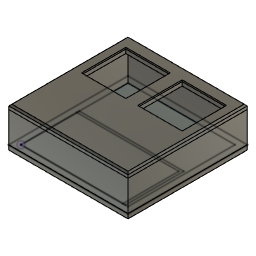
Keypad_Nogap_V2.5L (Autodesk Fusion 360 design; units mm, degrees)
Autodesk Fusion 360 part; units mm, degrees
sketch "Sketch1" plane through (0, 0, 0) normal (0, 0, 1) x (1, 0, 0) in component "case"
  line L0 (0, 0) -> (33.33, 0)
  line L1 (33.33, 0) -> (33.33, 18.3)
  line L2 (33.33, 18.3) -> (0, 18.3)
  line L3 (0, 18.3) -> (0, 0)
  line L4 (34.13, 0) -> (34.13, 19.1)
  line L5 (34.13, 19.1) -> (0, 19.1)
  line L6 (34.13, 0) -> (33.33, 0)
  line L7 (0, 19.1) -> (0, 18.3)
  line L8 (0, 0) -> (35, 0)
  line L9 (35, 0) -> (35, 35)
  line L10 (35, 35) -> (0, 35)
  line L11 (0, 35) -> (0, 0)
  line L12 (-2, 37) -> (-2, -2)
  line L13 (-2, -2) -> (37, -2)
  line L14 (37, -2) -> (37, 37)
  line L15 (37, 37) -> (-2, 37)
  dimension "d1" = 33.33
  dimension "d2" = 18.3
  dimension "d3" = 0.8
  dimension "d4" = 35
  dimension "d5" = 35
  dimension "d6" = 2
  constraint horizontal L0
  constraint vertical L1
  constraint horizontal L2
  constraint vertical L3
  constraint coincident L0.start L3.end
  constraint perpendicular L1 L6
  constraint perpendicular L2 L7
  constraint horizontal L8
  constraint vertical L9
  constraint horizontal L10
  constraint vertical L11
  measures "d1" distance of L0.start L0.end
  measures "d2" distance of L0.start L2.end
  measures "d4" distance of L0.start L8.end
  measures "d5" distance of L0.start L10.end
extrude "Extrude1" add sketch "Sketch1" against normal blind 2 contours L0 L1 L2 L3 L8 L11 | L1 L2 L4 L5 L6 L7 L8 L11 | L4 L5 L8 L9 L10 L11 | L12 L13 L14 L15 makes body 1 in component "case"
extrude "Extrude2" add sketch "Sketch1" along normal blind 1.7 contours L1 L2 L4 L5 L6 L7 L8 L11 bodies 1 in component "case"
ref_plane "WorkPlane1" through (17.5, 17.5, 1.7) normal (0, 0, 1) x (1, 0, 0) in component "case"
extrude "Extrude3" add sketch "Sketch1" along normal blind 10 bodies 1 in component "case"
chamfer "Chamfer1" distance 0.5 angle 45 2 edges at (17.065, 19.1, 0) (34.13, 9.55, 0) on bodies 1 in component "case"
sketch "Sketch2" plane through (17.5, 17.5, 1.7) normal (0, 0, 1) x (1, 0, 0) in component "case"
  line L0 (-17.5, -17.5) -> (15.83, -17.5)
  line L1 (15.83, -17.5) -> (15.83, 0.8)
  line L2 (15.83, 0.8) -> (-17.5, 0.8)
  line L3 (-17.5, 0.8) -> (-17.5, -17.5)
  line L4 (-17.5, -17.5) -> (-17.5, -12.25) construction
  line L5 (-17.5, -12.25) -> (-20, -12.25)
  line L6 (-20, -12.25) -> (-20, -4.75)
  line L7 (-20, -4.75) -> (-17.5, -4.75)
  line L8 (-17.5, -4.75) -> (-17.5, -12.25)
  dimension "d15" = 5.25
  dimension "d16" = 2.5
  dimension "d17" = 7.5
  constraint coincident L0.start L3.end
  constraint perpendicular L0 L4
  constraint horizontal L5
  constraint vertical L6
  constraint horizontal L7
  constraint vertical L8
  measures "d15" distance of L0.start L4.end
  measures "d16" distance of L4.end L5.end
  measures "d17" distance of L4.end L7.end
extrude "Extrude4" cut sketch "Sketch2" along normal blind 2.6 and the other way blind 0.1 contours L3 L5 L6 L7 L8 bodies 1 in component "case"
chamfer "Chamfer2" distance 1 angle 45 2 edges at (-1, 12.75, 1.6) (-1, 5.25, 1.6) on bodies 1 in component "case"
sketch "Sketch3" plane through (-2, 0, 0) normal (-1, 0, 0) x (0, -1, 0) in component "case"
  line L0 (-6.25, 1.6) -> (-11.75, 1.6)
  line L1 (-11.75, 1.6) -> (-12.75, 2.6)
  line L2 (-12.75, 2.6) -> (-12.75, 4.3)
  line L3 (-12.75, 4.3) -> (-5.25, 4.3)
  line L4 (-5.25, 4.3) -> (-5.25, 2.6)
  line L5 (-5.25, 2.6) -> (-6.25, 1.6)
  line L6 (-37, 10) -> (-37, -2)
  line L7 (-37, -2) -> (2, -2)
  line L8 (2, -2) -> (2, 10)
  line L9 (2, 10) -> (-37, 10)
  line L10 (-4.25, 2.1858) -> (-5.8358, 0.6)
  line L11 (-5.8358, 0.6) -> (-12.1642, 0.6)
  line L12 (-12.1642, 0.6) -> (-13.75, 2.1858)
  line L13 (-13.75, 2.1858) -> (-13.75, 5.3)
  line L14 (-13.75, 5.3) -> (-4.25, 5.3)
  line L15 (-4.25, 5.3) -> (-4.25, 2.1858)
  dimension "d23" = -1
  measures "d23" distance of L5
extrude "Extrude5" cut sketch "Sketch3" against normal blind 0.5 contours L10 L11 L12 L13 L14 L15 bodies 1 in component "case"
fillet "Fillet1" radius 0.5 12 edges at (-1.5, 12.9571, 1.3929) (-2, 12.9571, 1.3929) (-2, 13.75, 3.7429) (-1.5, 13.75, 3.7429) (-1.5, 9, 0.6) (-2, 9, 0.6) (-1.5, 9, 5.3) (-2, 9, 5.3) (-1.5, 4.25, 3.7429) (-2, 4.25, 3.7429) (-1.5, 5.0429, 1.3929) (-2, 5.0429, 1.3929) on bodies 1 in component "case"
sketch "Sketch4" plane through (0, 0, 10) normal (0, 0, 1) x (-1, 0, 0) in component "case"
  line L0 (0, 0) -> (0, -35)
  line L1 (0, -35) -> (-35, -35)
  line L2 (-35, -35) -> (-35, 0)
  line L3 (-35, 0) -> (0, 0)
  line L4 (-37, -37) -> (2, -37)
  line L5 (2, -37) -> (2, 2)
  line L6 (2, 2) -> (-37, 2)
  line L7 (-37, 2) -> (-37, -37)
  line L8 (0.8, 0.8) -> (0.8, -35.8)
  line L9 (0.8, -35.8) -> (-35.8, -35.8)
  line L10 (-35.8, -35.8) -> (-35.8, 0.8)
  line L11 (-35.8, 0.8) -> (0.8, 0.8)
  dimension "d28" = -0.8
extrude "Extrude6" cut sketch "Sketch4" against normal blind 1 contours L8 L9 L10 L11 bodies 1 in component "case"
sketch "Sketch1 (2)" plane through (0, 0, 10) normal (0, 0, 1) x (-1, 0, 0) in component "lid"
  line L0 (0.8, -35.8) -> (-35.8, -35.8)
  line L1 (-35.8, -35.8) -> (-35.8, 0.8)
  line L2 (-35.8, 0.8) -> (0.8, 0.8)
  line L3 (0.8, 0.8) -> (0.8, -35.8)
  line L4 (-37, -37) -> (2, -37)
  line L5 (2, -37) -> (2, 2)
  line L6 (2, 2) -> (-37, 2)
  line L7 (-37, 2) -> (-37, -37)
  line L8 (-35, -35) -> (-35, 0)
  line L9 (-35, 0) -> (0, 0)
  line L10 (0, 0) -> (0, -35)
  line L11 (0, -35) -> (-35, -35)
  line L12 (-35.8, 0.8) -> (-35.8, -35.8)
  line L13 (-35.8, -35.8) -> (0.8, -35.8)
  line L14 (0.8, -35.8) -> (0.8, 0.8)
  line L15 (0.8, 0.8) -> (-35.8, 0.8)
  line L16 (0.7, 0.7) -> (0.7, -35.7)
  line L17 (0.7, -35.7) -> (-35.7, -35.7)
  line L18 (-35.7, -35.7) -> (-35.7, 0.7)
  line L19 (-35.7, 0.7) -> (0.7, 0.7)
  dimension "d31" = 0.1
extrude "Extrude1'" add sketch "Sketch1 (2)" against normal blind 0.9 separate body contours L16 L17 L18 L19 makes body 2 in component "lid"
sketch "Sketch2 (2)" plane through (0, 0, 10) normal (0, 0, 1) x (-1, 0, 0) in component "lid"
  line L0 (0.8, -35.8) -> (-35.8, -35.8)
  line L1 (-35.8, -35.8) -> (-35.8, 0.8)
  line L2 (-35.8, 0.8) -> (0.8, 0.8)
  line L3 (0.8, 0.8) -> (0.8, -35.8)
  line L4 (-37, -37) -> (2, -37)
  line L5 (2, -37) -> (2, 2)
  line L6 (2, 2) -> (-37, 2)
  line L7 (-37, 2) -> (-37, -37)
  line L8 (-37, -37) -> (2, -37)
  line L9 (2, -37) -> (2, 2)
  line L10 (2, 2) -> (-37, 2)
  line L11 (-37, 2) -> (-37, -37)
  constraint horizontal L8
  constraint vertical L9
  constraint horizontal L10
  constraint vertical L11
  constraint coincident L5.end L6.start
  constraint coincident L4.start L7.end
extrude "Extrude2'" add sketch "Sketch2 (2)" along normal blind 1.5 contours L0 L1 L2 L3 | L4 L5 L6 L7 L8 L9 L10 L11 bodies 2 in component "lid"
sketch "Sketch3 (2)" plane through (0, 0, 11.5) normal (0, 0, 1) x (-1, 0, 0) in component "lid"
  line L0 (-37, 2) -> (-37, -37)
  line L1 (-37, -37) -> (2, -37)
  line L2 (2, -37) -> (2, 2)
  line L3 (2, 2) -> (-37, 2)
  line L4 (-1.2835, -33) -> (-15.2835, -33)
  line L5 (-15.2835, -33) -> (-15.2835, -19)
  line L6 (-15.2835, -19) -> (-1.2835, -19)
  line L7 (-1.2835, -19) -> (-1.2835, -33)
  line L8 (-15.2835, -19) -> (-19.7168, -19) construction
  line L9 (-19.7168, -19) -> (-33.7168, -19)
  line L10 (-33.7168, -19) -> (-33.7168, -33)
  line L11 (-33.7168, -33) -> (-19.7168, -33)
  line L12 (-19.7168, -33) -> (-19.7168, -19)
  line L13 (-35, -35) -> (-35, 0)
  line L14 (-35, 0) -> (0, 0)
  line L15 (0, 0) -> (0, -35)
  line L16 (0, -35) -> (-35, -35)
  line L17 (-35.8, 0.8) -> (-35.8, -35.8)
  line L18 (-35.8, -35.8) -> (0.8, -35.8)
  line L19 (0.8, -35.8) -> (0.8, 0.8)
  line L20 (0.8, 0.8) -> (-35.8, 0.8)
  line L21 (0.8, -35.8) -> (-35.8, -35.8)
  line L22 (-35.8, -35.8) -> (-35.8, 0.8)
  line L23 (-35.8, 0.8) -> (0.8, 0.8)
  line L24 (0.8, 0.8) -> (0.8, -35.8)
  line L25 (-37, -37) -> (2, -37)
  line L26 (2, -37) -> (2, 2)
  line L27 (2, 2) -> (-37, 2)
  line L28 (-37, 2) -> (-37, -37)
  line L29 (0.8, -26.6121) -> (-1.2835, -26.6121) construction
  line L30 (-6.7358, -33) -> (-6.7358, -35) construction
  dimension "d36" = 14
  dimension "d37" = 14
  dimension "d38" = 4.4333
  dimension "d39" = 14
  dimension "d40" = 14
  dimension "d45" = 2.0835
  constraint horizontal L4
  constraint vertical L5
  constraint horizontal L6
  constraint vertical L7
  constraint perpendicular L5 L8
  constraint horizontal L9
  constraint vertical L10
  constraint horizontal L11
  constraint vertical L12
  constraint coincident L24 L29.start
  constraint coincident L7 L29.end
  constraint perpendicular L7 L29
  constraint coincident L4 L30.start
  constraint coincident L16 L30.end
  constraint perpendicular L16 L30
  measures "d36" distance of L4.start L4.end
  measures "d37" distance of L4.start L6.end
  measures "d38" distance of L5.end L8.end
  measures "d39" distance of L8.end L9.end
  measures "d40" distance of L8.end L11.end
  measures "d45" distance of L29.start L29.end
extrude "Extrude3'" cut sketch "Sketch3 (2)" against normal blind 2 contours L4 L5 L6 L7 | L9 L10 L11 L12 bodies 2 in component "lid"
chamfer "Chamfer1'" distance 0.5 angle 45 4 edges at (37, 17.5, 11.5) (17.5, -2, 11.5) (-2, 17.5, 11.5) (17.5, 37, 11.5) on bodies 2 in component "lid"
chamfer "Chamfer2'" distance 0.25 angle 45 8 edges at (26.7168, 33, 11.5) (15.2835, 26, 11.5) (8.2835, 33, 11.5) (1.2835, 26, 11.5) (8.2835, 19, 11.5) (26.7168, 19, 11.5) (19.7168, 26, 11.5) (33.7168, 26, 11.5) on bodies 2 in component "lid"
chamfer "Chamfer3" distance 0.5 angle 45 4 edges at (37, 17.5, -2) (17.5, -2, -2) (-2, 17.5, -2) (17.5, 37, -2) on bodies 1 in component "case"
component "case" placed x (1, 0, 0) y (0, 1, 0) z (0, 0, 1) at (0, 0, 0)
component "lid" placed x (1, 0, 0) y (0, 1, 0) z (0, 0, 1) at (0, 0, 0)
